Autodesk Fusion 360 part; units mm, degrees
(part 2 of 2)
  line L915 (6.2451, -45) -> (4.5882, -45)
  line L916 (6.2451, 10) -> (4.5882, 10)
  line L917 (3.4167, -7.8284) -> (4.5882, -9)
  line L918 (4.5882, -50) -> (3.4167, -51.1716)
  line L919 (7.4167, -36.1716) -> (6.2451, -35)
  line L920 (3.4167, 13.8284) -> (3.4167, 12.1716)
  line L921 (6.2451, -9) -> (7.4167, -7.8284)
  line L922 (4.5882, -20) -> (3.4167, -21.1716)
  line L923 (4.5882, -10) -> (3.4167, -11.1716)
  line L924 (3.4167, -41.1716) -> (3.4167, -42.8284)
  line L925 (3.4167, 7.1716) -> (4.5882, 6)
  line L926 (4.5882, -15) -> (3.4167, -16.1716)
  line L927 (3.4167, -32.8284) -> (4.5882, -34)
  line L928 (3.4167, -42.8284) -> (4.5882, -44)
  line L929 (6.2451, -25) -> (4.5882, -25)
  line L930 (3.4167, -47.8284) -> (4.5882, -49)
  line L931 (7.4167, -26.1716) -> (6.2451, -25)
  line L932 (4.5882, -39) -> (6.2451, -39)
  line L933 (6.2451, 0) -> (4.5882, 0)
  line L934 (4.5882, 15) -> (3.4167, 13.8284)
  line L935 (3.4167, -37.8284) -> (4.5882, -39)
  line L936 (6.2451, -20) -> (4.5882, -20)
  line L937 (4.5882, 11) -> (6.2451, 11)
  line L938 (7.4167, -11.1716) -> (6.2451, -10)
  line L939 (3.4167, -27.8284) -> (4.5882, -29)
  line L940 (4.5882, 10) -> (3.4167, 8.8284)
  line L941 (6.2451, 11) -> (7.4167, 12.1716)
  line L942 (7.4167, -1.1716) -> (6.2451, 0)
  line L943 (6.2451, -39) -> (7.4167, -37.8284)
  line L944 (4.5882, -45) -> (3.4167, -46.1716)
  line L945 (7.4167, -22.8284) -> (7.4167, -21.1716)
  line L946 (3.4167, -26.1716) -> (3.4167, -27.8284)
  line L947 (3.4167, -16.1716) -> (3.4167, -17.8284)
  line L948 (6.2451, -54) -> (7.4167, -52.8284)
  line L949 (7.4167, -16.1716) -> (6.2451, -15)
  line L950 (3.4167, -11.1716) -> (3.4167, -12.8284)
  line L951 (4.5882, -40) -> (3.4167, -41.1716)
  line L952 (3.4167, -2.8284) -> (4.5882, -4)
  line L953 (3.4167, -12.8284) -> (4.5882, -14)
  line L954 (3.4167, 3.8284) -> (3.4167, 2.1716)
  line L955 (7.4167, -37.8284) -> (7.4167, -36.1716)
  line L956 (7.4167, -52.8284) -> (7.4167, -51.1716)
  line L957 (7.4167, -42.8284) -> (7.4167, -41.1716)
  line L958 (7.4167, 3.8284) -> (6.2451, 5)
  line L959 (6.2451, -5) -> (4.5882, -5)
  line L960 (7.4167, -51.1716) -> (6.2451, -50)
  line L961 (4.5882, -30) -> (3.4167, -31.1716)
  line L962 (4.5882, -4) -> (6.2451, -4)
  line L963 (7.4167, 7.1716) -> (7.4167, 8.8284)
  line L964 (4.5882, -34) -> (6.2451, -34)
  line L965 (6.2451, -15) -> (4.5882, -15)
  line L966 (7.4167, 2.1716) -> (7.4167, 3.8284)
  line L967 (6.2451, 20) -> (4.5882, 20)
  line L968 (4.5882, -54) -> (6.2451, -54)
  line L969 (3.4167, 12.1716) -> (4.5882, 11)
  line L970 (3.4167, -36.1716) -> (3.4167, -37.8284)
  line L971 (7.4167, -41.1716) -> (6.2451, -40)
  line L972 (7.4167, 13.8284) -> (6.2451, 15)
  line L973 (7.4167, 18.8284) -> (6.2451, 20)
  line L974 (7.4167, -7.8284) -> (7.4167, -6.1716)
  line L975 (6.2451, -29) -> (7.4167, -27.8284)
  line L976 (8.3333, -6.1716) -> (8.3333, -7.8284)
  line L977 (11.1618, -40) -> (9.5049, -40)
  line L978 (12.3333, -27.8284) -> (12.3333, -26.1716)
  line L979 (9.5049, 5) -> (8.3333, 3.8284)
  line L980 (8.3333, -31.1716) -> (8.3333, -32.8284)
  line L981 (12.3333, -2.8284) -> (12.3333, -1.1716)
  line L982 (9.5049, 20) -> (8.3333, 18.8284)
  line L983 (8.3333, 2.1716) -> (9.5049, 1)
  line L984 (8.3333, -1.1716) -> (8.3333, -2.8284)
  line L985 (8.3333, 18.8284) -> (8.3333, 17.1716)
  line L986 (9.5049, -29) -> (11.1618, -29)
  line L987 (11.1618, -49) -> (12.3333, -47.8284)
  line L988 (11.1618, 5) -> (9.5049, 5)
  line L989 (11.1618, -24) -> (12.3333, -22.8284)
  line L990 (8.3333, -51.1716) -> (8.3333, -52.8284)
  line L991 (12.3333, -6.1716) -> (11.1618, -5)
  line L992 (12.3333, -47.8284) -> (12.3333, -46.1716)
  line L993 (12.3333, -32.8284) -> (12.3333, -31.1716)
  line L994 (12.3333, 8.8284) -> (11.1618, 10)
  line L995 (8.3333, 17.1716) -> (9.5049, 16)
  line L996 (9.5049, -9) -> (11.1618, -9)
  line L997 (12.3333, -46.1716) -> (11.1618, -45)
  line L998 (11.1618, 16) -> (12.3333, 17.1716)
  line L999 (11.1618, -44) -> (12.3333, -42.8284)
  line L1000 (9.5049, -14) -> (11.1618, -14)
  line L1001 (11.1618, 6) -> (12.3333, 7.1716)
  line L1002 (9.5049, -49) -> (11.1618, -49)
  line L1003 (9.5049, -44) -> (11.1618, -44)
  line L1004 (12.3333, -21.1716) -> (11.1618, -20)
  line L1005 (9.5049, 1) -> (11.1618, 1)
  line L1006 (11.1618, -4) -> (12.3333, -2.8284)
  line L1007 (12.3333, -17.8284) -> (12.3333, -16.1716)
  line L1008 (11.1618, -30) -> (9.5049, -30)
  line L1009 (9.5049, -5) -> (8.3333, -6.1716)
  line L1010 (11.1618, -19) -> (12.3333, -17.8284)
  line L1011 (11.1618, -14) -> (12.3333, -12.8284)
  line L1012 (8.3333, -22.8284) -> (9.5049, -24)
  line L1013 (11.1618, -34) -> (12.3333, -32.8284)
  line L1014 (12.3333, -31.1716) -> (11.1618, -30)
  line L1015 (12.3333, -12.8284) -> (12.3333, -11.1716)
  line L1016 (8.3333, -21.1716) -> (8.3333, -22.8284)
  line L1017 (9.5049, -35) -> (8.3333, -36.1716)
  line L1018 (9.5049, 0) -> (8.3333, -1.1716)
  line L1019 (8.3333, -52.8284) -> (9.5049, -54)
  line L1020 (11.1618, -10) -> (9.5049, -10)
  line L1021 (11.1618, 1) -> (12.3333, 2.1716)
  line L1022 (8.3333, -17.8284) -> (9.5049, -19)
  line L1023 (8.3333, -46.1716) -> (8.3333, -47.8284)
  line L1024 (12.3333, 17.1716) -> (12.3333, 18.8284)
  line L1025 (9.5049, -19) -> (11.1618, -19)
  line L1026 (9.5049, 16) -> (11.1618, 16)
  line L1027 (9.5049, 6) -> (11.1618, 6)
  line L1028 (9.5049, -24) -> (11.1618, -24)
  line L1029 (9.5049, -25) -> (8.3333, -26.1716)
  line L1030 (11.1618, -35) -> (9.5049, -35)
  line L1031 (12.3333, 12.1716) -> (12.3333, 13.8284)
  line L1032 (11.1618, -50) -> (9.5049, -50)
  line L1033 (8.3333, 8.8284) -> (8.3333, 7.1716)
  line L1034 (11.1618, 15) -> (9.5049, 15)
  line L1035 (11.1618, -45) -> (9.5049, -45)
  line L1036 (11.1618, 10) -> (9.5049, 10)
  line L1037 (8.3333, -7.8284) -> (9.5049, -9)
  line L1038 (9.5049, -50) -> (8.3333, -51.1716)
  line L1039 (12.3333, -36.1716) -> (11.1618, -35)
  line L1040 (8.3333, 13.8284) -> (8.3333, 12.1716)
  line L1041 (11.1618, -9) -> (12.3333, -7.8284)
  line L1042 (9.5049, -20) -> (8.3333, -21.1716)
  line L1043 (9.5049, -10) -> (8.3333, -11.1716)
  line L1044 (8.3333, -41.1716) -> (8.3333, -42.8284)
  line L1045 (8.3333, 7.1716) -> (9.5049, 6)
  line L1046 (9.5049, -15) -> (8.3333, -16.1716)
  line L1047 (8.3333, -32.8284) -> (9.5049, -34)
  line L1048 (8.3333, -42.8284) -> (9.5049, -44)
  line L1049 (11.1618, -25) -> (9.5049, -25)
  line L1050 (8.3333, -47.8284) -> (9.5049, -49)
  line L1051 (12.3333, -26.1716) -> (11.1618, -25)
  line L1052 (9.5049, -39) -> (11.1618, -39)
  line L1053 (11.1618, 0) -> (9.5049, 0)
  line L1054 (9.5049, 15) -> (8.3333, 13.8284)
  line L1055 (8.3333, -37.8284) -> (9.5049, -39)
  line L1056 (11.1618, -20) -> (9.5049, -20)
  line L1057 (9.5049, 11) -> (11.1618, 11)
  line L1058 (12.3333, -11.1716) -> (11.1618, -10)
  line L1059 (8.3333, -27.8284) -> (9.5049, -29)
  line L1060 (9.5049, 10) -> (8.3333, 8.8284)
  line L1061 (11.1618, 11) -> (12.3333, 12.1716)
  line L1062 (12.3333, -1.1716) -> (11.1618, 0)
  line L1063 (11.1618, -39) -> (12.3333, -37.8284)
  line L1064 (9.5049, -45) -> (8.3333, -46.1716)
  line L1065 (12.3333, -22.8284) -> (12.3333, -21.1716)
  line L1066 (8.3333, -26.1716) -> (8.3333, -27.8284)
  line L1067 (8.3333, -16.1716) -> (8.3333, -17.8284)
  line L1068 (11.1618, -54) -> (12.3333, -52.8284)
  line L1069 (12.3333, -16.1716) -> (11.1618, -15)
  line L1070 (8.3333, -11.1716) -> (8.3333, -12.8284)
  line L1071 (9.5049, -40) -> (8.3333, -41.1716)
  line L1072 (8.3333, -2.8284) -> (9.5049, -4)
  line L1073 (8.3333, -12.8284) -> (9.5049, -14)
  line L1074 (8.3333, 3.8284) -> (8.3333, 2.1716)
  line L1075 (12.3333, -37.8284) -> (12.3333, -36.1716)
  line L1076 (12.3333, -52.8284) -> (12.3333, -51.1716)
  line L1077 (12.3333, -42.8284) -> (12.3333, -41.1716)
  line L1078 (12.3333, 3.8284) -> (11.1618, 5)
  line L1079 (11.1618, -5) -> (9.5049, -5)
  line L1080 (12.3333, -51.1716) -> (11.1618, -50)
  line L1081 (9.5049, -30) -> (8.3333, -31.1716)
  line L1082 (9.5049, -4) -> (11.1618, -4)
  line L1083 (12.3333, 7.1716) -> (12.3333, 8.8284)
  line L1084 (9.5049, -34) -> (11.1618, -34)
  line L1085 (11.1618, -15) -> (9.5049, -15)
  line L1086 (12.3333, 2.1716) -> (12.3333, 3.8284)
  line L1087 (11.1618, 20) -> (9.5049, 20)
  line L1088 (9.5049, -54) -> (11.1618, -54)
  line L1089 (8.3333, 12.1716) -> (9.5049, 11)
  line L1090 (8.3333, -36.1716) -> (8.3333, -37.8284)
  line L1091 (12.3333, -41.1716) -> (11.1618, -40)
  line L1092 (12.3333, 13.8284) -> (11.1618, 15)
  line L1093 (12.3333, 18.8284) -> (11.1618, 20)
  line L1094 (12.3333, -7.8284) -> (12.3333, -6.1716)
  line L1095 (11.1618, -29) -> (12.3333, -27.8284)
  line L1096 (13.25, -6.1716) -> (13.25, -7.8284)
  line L1097 (16.0784, -40) -> (14.4216, -40)
  line L1098 (17.25, -27.8284) -> (17.25, -26.1716)
  line L1099 (14.4216, 5) -> (13.25, 3.8284)
  line L1100 (13.25, -31.1716) -> (13.25, -32.8284)
  line L1101 (17.25, -2.8284) -> (17.25, -1.1716)
  line L1102 (14.4216, 20) -> (13.25, 18.8284)
  line L1103 (13.25, 2.1716) -> (14.4216, 1)
  line L1104 (13.25, -1.1716) -> (13.25, -2.8284)
  line L1105 (13.25, 18.8284) -> (13.25, 17.1716)
  line L1106 (14.4216, -29) -> (16.0784, -29)
  line L1107 (16.0784, -49) -> (17.25, -47.8284)
  line L1108 (16.0784, 5) -> (14.4216, 5)
  line L1109 (16.0784, -24) -> (17.25, -22.8284)
  line L1110 (13.25, -51.1716) -> (13.25, -52.8284)
  line L1111 (17.25, -6.1716) -> (16.0784, -5)
  line L1112 (17.25, -47.8284) -> (17.25, -46.1716)
  line L1113 (17.25, -32.8284) -> (17.25, -31.1716)
  line L1114 (17.25, 8.8284) -> (16.0784, 10)
  line L1115 (13.25, 17.1716) -> (14.4216, 16)
  line L1116 (14.4216, -9) -> (16.0784, -9)
  line L1117 (17.25, -46.1716) -> (16.0784, -45)
  line L1118 (16.0784, 16) -> (17.25, 17.1716)
  line L1119 (16.0784, -44) -> (17.25, -42.8284)
  line L1120 (14.4216, -14) -> (16.0784, -14)
  line L1121 (16.0784, 6) -> (17.25, 7.1716)
  line L1122 (14.4216, -49) -> (16.0784, -49)
  line L1123 (14.4216, -44) -> (16.0784, -44)
  line L1124 (17.25, -21.1716) -> (16.0784, -20)
  line L1125 (14.4216, 1) -> (16.0784, 1)
  line L1126 (16.0784, -4) -> (17.25, -2.8284)
  line L1127 (17.25, -17.8284) -> (17.25, -16.1716)
  line L1128 (16.0784, -30) -> (14.4216, -30)
  line L1129 (14.4216, -5) -> (13.25, -6.1716)
  line L1130 (16.0784, -19) -> (17.25, -17.8284)
  line L1131 (16.0784, -14) -> (17.25, -12.8284)
  line L1132 (13.25, -22.8284) -> (14.4216, -24)
  line L1133 (16.0784, -34) -> (17.25, -32.8284)
  line L1134 (17.25, -31.1716) -> (16.0784, -30)
  line L1135 (17.25, -12.8284) -> (17.25, -11.1716)
  line L1136 (13.25, -21.1716) -> (13.25, -22.8284)
  line L1137 (14.4216, -35) -> (13.25, -36.1716)
  line L1138 (14.4216, 0) -> (13.25, -1.1716)
  line L1139 (13.25, -52.8284) -> (14.4216, -54)
  line L1140 (16.0784, -10) -> (14.4216, -10)
  line L1141 (16.0784, 1) -> (17.25, 2.1716)
  line L1142 (13.25, -17.8284) -> (14.4216, -19)
  line L1143 (13.25, -46.1716) -> (13.25, -47.8284)
  line L1144 (17.25, 17.1716) -> (17.25, 18.8284)
  line L1145 (14.4216, -19) -> (16.0784, -19)
  line L1146 (14.4216, 16) -> (16.0784, 16)
  line L1147 (14.4216, 6) -> (16.0784, 6)
  line L1148 (14.4216, -24) -> (16.0784, -24)
  line L1149 (14.4216, -25) -> (13.25, -26.1716)
  line L1150 (16.0784, -35) -> (14.4216, -35)
  line L1151 (17.25, 12.1716) -> (17.25, 13.8284)
  line L1152 (16.0784, -50) -> (14.4216, -50)
  line L1153 (13.25, 8.8284) -> (13.25, 7.1716)
  line L1154 (16.0784, 15) -> (14.4216, 15)
  line L1155 (16.0784, -45) -> (14.4216, -45)
  line L1156 (16.0784, 10) -> (14.4216, 10)
  line L1157 (13.25, -7.8284) -> (14.4216, -9)
  line L1158 (14.4216, -50) -> (13.25, -51.1716)
  line L1159 (17.25, -36.1716) -> (16.0784, -35)
  line L1160 (13.25, 13.8284) -> (13.25, 12.1716)
  line L1161 (16.0784, -9) -> (17.25, -7.8284)
  line L1162 (14.4216, -20) -> (13.25, -21.1716)
  line L1163 (14.4216, -10) -> (13.25, -11.1716)
  line L1164 (13.25, -41.1716) -> (13.25, -42.8284)
  line L1165 (13.25, 7.1716) -> (14.4216, 6)
  line L1166 (14.4216, -15) -> (13.25, -16.1716)
  line L1167 (13.25, -32.8284) -> (14.4216, -34)
  line L1168 (13.25, -42.8284) -> (14.4216, -44)
  line L1169 (16.0784, -25) -> (14.4216, -25)
  line L1170 (13.25, -47.8284) -> (14.4216, -49)
  line L1171 (17.25, -26.1716) -> (16.0784, -25)
  line L1172 (14.4216, -39) -> (16.0784, -39)
  line L1173 (16.0784, 0) -> (14.4216, 0)
  line L1174 (14.4216, 15) -> (13.25, 13.8284)
  line L1175 (13.25, -37.8284) -> (14.4216, -39)
  line L1176 (16.0784, -20) -> (14.4216, -20)
  line L1177 (14.4216, 11) -> (16.0784, 11)
  line L1178 (17.25, -11.1716) -> (16.0784, -10)
  line L1179 (13.25, -27.8284) -> (14.4216, -29)
  line L1180 (14.4216, 10) -> (13.25, 8.8284)
  line L1181 (16.0784, 11) -> (17.25, 12.1716)
  line L1182 (17.25, -1.1716) -> (16.0784, 0)
  line L1183 (16.0784, -39) -> (17.25, -37.8284)
  line L1184 (14.4216, -45) -> (13.25, -46.1716)
  line L1185 (17.25, -22.8284) -> (17.25, -21.1716)
  line L1186 (13.25, -26.1716) -> (13.25, -27.8284)
  line L1187 (13.25, -16.1716) -> (13.25, -17.8284)
  line L1188 (16.0784, -54) -> (17.25, -52.8284)
  line L1189 (17.25, -16.1716) -> (16.0784, -15)
  line L1190 (13.25, -11.1716) -> (13.25, -12.8284)
  line L1191 (14.4216, -40) -> (13.25, -41.1716)
  line L1192 (13.25, -2.8284) -> (14.4216, -4)
  line L1193 (13.25, -12.8284) -> (14.4216, -14)
  line L1194 (13.25, 3.8284) -> (13.25, 2.1716)
  line L1195 (17.25, -37.8284) -> (17.25, -36.1716)
  line L1196 (17.25, -52.8284) -> (17.25, -51.1716)
  line L1197 (17.25, -42.8284) -> (17.25, -41.1716)
  line L1198 (17.25, 3.8284) -> (16.0784, 5)
  line L1199 (16.0784, -5) -> (14.4216, -5)
  line L1200 (17.25, -51.1716) -> (16.0784, -50)
  line L1201 (14.4216, -30) -> (13.25, -31.1716)
  line L1202 (14.4216, -4) -> (16.0784, -4)
  line L1203 (17.25, 7.1716) -> (17.25, 8.8284)
  line L1204 (14.4216, -34) -> (16.0784, -34)
  line L1205 (16.0784, -15) -> (14.4216, -15)
  line L1206 (17.25, 2.1716) -> (17.25, 3.8284)
  line L1207 (16.0784, 20) -> (14.4216, 20)
  line L1208 (14.4216, -54) -> (16.0784, -54)
  line L1209 (13.25, 12.1716) -> (14.4216, 11)
  line L1210 (13.25, -36.1716) -> (13.25, -37.8284)
  line L1211 (17.25, -41.1716) -> (16.0784, -40)
  line L1212 (17.25, 13.8284) -> (16.0784, 15)
  line L1213 (17.25, 18.8284) -> (16.0784, 20)
  line L1214 (17.25, -7.8284) -> (17.25, -6.1716)
  line L1215 (16.0784, -29) -> (17.25, -27.8284)
  line L1216 (18.1667, -6.1716) -> (18.1667, -7.8284)
  line L1217 (20.9951, -40) -> (19.3382, -40)
  line L1218 (22.1667, -27.8284) -> (22.1667, -26.1716)
  line L1219 (19.3382, 5) -> (18.1667, 3.8284)
  line L1220 (18.1667, -31.1716) -> (18.1667, -32.8284)
  line L1221 (22.1667, -2.8284) -> (22.1667, -1.1716)
  line L1222 (19.3382, 20) -> (18.1667, 18.8284)
  line L1223 (18.1667, 2.1716) -> (19.3382, 1)
  line L1224 (18.1667, -1.1716) -> (18.1667, -2.8284)
  line L1225 (18.1667, 18.8284) -> (18.1667, 17.1716)
  line L1226 (19.3382, -29) -> (20.9951, -29)
  line L1227 (20.9951, -49) -> (22.1667, -47.8284)
  line L1228 (20.9951, 5) -> (19.3382, 5)
  line L1229 (20.9951, -24) -> (22.1667, -22.8284)
  line L1230 (18.1667, -51.1716) -> (18.1667, -52.8284)
  line L1231 (22.1667, -6.1716) -> (20.9951, -5)
  line L1232 (22.1667, -47.8284) -> (22.1667, -46.1716)
  line L1233 (22.1667, -32.8284) -> (22.1667, -31.1716)
  line L1234 (22.1667, 8.8284) -> (20.9951, 10)
  line L1235 (18.1667, 17.1716) -> (19.3382, 16)
  line L1236 (19.3382, -9) -> (20.9951, -9)
  line L1237 (22.1667, -46.1716) -> (20.9951, -45)
  line L1238 (20.9951, 16) -> (22.1667, 17.1716)
  line L1239 (20.9951, -44) -> (22.1667, -42.8284)
  line L1240 (19.3382, -14) -> (20.9951, -14)
  line L1241 (20.9951, 6) -> (22.1667, 7.1716)
  line L1242 (19.3382, -49) -> (20.9951, -49)
  line L1243 (19.3382, -44) -> (20.9951, -44)
  line L1244 (22.1667, -21.1716) -> (20.9951, -20)
  line L1245 (19.3382, 1) -> (20.9951, 1)
  line L1246 (20.9951, -4) -> (22.1667, -2.8284)
  line L1247 (22.1667, -17.8284) -> (22.1667, -16.1716)
  line L1248 (20.9951, -30) -> (19.3382, -30)
  line L1249 (19.3382, -5) -> (18.1667, -6.1716)
  line L1250 (20.9951, -19) -> (22.1667, -17.8284)
  line L1251 (20.9951, -14) -> (22.1667, -12.8284)
  line L1252 (18.1667, -22.8284) -> (19.3382, -24)
  line L1253 (20.9951, -34) -> (22.1667, -32.8284)
  line L1254 (22.1667, -31.1716) -> (20.9951, -30)
  line L1255 (22.1667, -12.8284) -> (22.1667, -11.1716)
  line L1256 (18.1667, -21.1716) -> (18.1667, -22.8284)
  line L1257 (19.3382, -35) -> (18.1667, -36.1716)
  line L1258 (19.3382, 0) -> (18.1667, -1.1716)
  line L1259 (18.1667, -52.8284) -> (19.3382, -54)
  line L1260 (20.9951, -10) -> (19.3382, -10)
  line L1261 (20.9951, 1) -> (22.1667, 2.1716)
  line L1262 (18.1667, -17.8284) -> (19.3382, -19)
  line L1263 (18.1667, -46.1716) -> (18.1667, -47.8284)
  line L1264 (22.1667, 17.1716) -> (22.1667, 18.8284)
  line L1265 (19.3382, -19) -> (20.9951, -19)
  line L1266 (19.3382, 16) -> (20.9951, 16)
  line L1267 (19.3382, 6) -> (20.9951, 6)
  line L1268 (19.3382, -24) -> (20.9951, -24)
  line L1269 (19.3382, -25) -> (18.1667, -26.1716)
  line L1270 (20.9951, -35) -> (19.3382, -35)
  line L1271 (22.1667, 12.1716) -> (22.1667, 13.8284)
  line L1272 (20.9951, -50) -> (19.3382, -50)
  line L1273 (18.1667, 8.8284) -> (18.1667, 7.1716)
  line L1274 (20.9951, 15) -> (19.3382, 15)
  line L1275 (20.9951, -45) -> (19.3382, -45)
  line L1276 (20.9951, 10) -> (19.3382, 10)
  line L1277 (18.1667, -7.8284) -> (19.3382, -9)
  line L1278 (19.3382, -50) -> (18.1667, -51.1716)
  line L1279 (22.1667, -36.1716) -> (20.9951, -35)
  line L1280 (18.1667, 13.8284) -> (18.1667, 12.1716)
  line L1281 (20.9951, -9) -> (22.1667, -7.8284)
  line L1282 (19.3382, -20) -> (18.1667, -21.1716)
  line L1283 (19.3382, -10) -> (18.1667, -11.1716)
  line L1284 (18.1667, -41.1716) -> (18.1667, -42.8284)
  line L1285 (18.1667, 7.1716) -> (19.3382, 6)
  line L1286 (19.3382, -15) -> (18.1667, -16.1716)
  line L1287 (18.1667, -32.8284) -> (19.3382, -34)
  line L1288 (18.1667, -42.8284) -> (19.3382, -44)
  line L1289 (20.9951, -25) -> (19.3382, -25)
  line L1290 (18.1667, -47.8284) -> (19.3382, -49)
  line L1291 (22.1667, -26.1716) -> (20.9951, -25)
  line L1292 (19.3382, -39) -> (20.9951, -39)
  line L1293 (20.9951, 0) -> (19.3382, 0)
  line L1294 (19.3382, 15) -> (18.1667, 13.8284)
  line L1295 (18.1667, -37.8284) -> (19.3382, -39)
  line L1296 (20.9951, -20) -> (19.3382, -20)
  line L1297 (19.3382, 11) -> (20.9951, 11)
  line L1298 (22.1667, -11.1716) -> (20.9951, -10)
  line L1299 (18.1667, -27.8284) -> (19.3382, -29)
  line L1300 (19.3382, 10) -> (18.1667, 8.8284)
  line L1301 (20.9951, 11) -> (22.1667, 12.1716)
  line L1302 (22.1667, -1.1716) -> (20.9951, 0)
  line L1303 (20.9951, -39) -> (22.1667, -37.8284)
  line L1304 (19.3382, -45) -> (18.1667, -46.1716)
  line L1305 (22.1667, -22.8284) -> (22.1667, -21.1716)
  line L1306 (18.1667, -26.1716) -> (18.1667, -27.8284)
  line L1307 (18.1667, -16.1716) -> (18.1667, -17.8284)
  line L1308 (20.9951, -54) -> (22.1667, -52.8284)
  line L1309 (22.1667, -16.1716) -> (20.9951, -15)
  line L1310 (18.1667, -11.1716) -> (18.1667, -12.8284)
  line L1311 (19.3382, -40) -> (18.1667, -41.1716)
  line L1312 (18.1667, -2.8284) -> (19.3382, -4)
  line L1313 (18.1667, -12.8284) -> (19.3382, -14)
  line L1314 (18.1667, 3.8284) -> (18.1667, 2.1716)
  line L1315 (22.1667, -37.8284) -> (22.1667, -36.1716)
  line L1316 (22.1667, -52.8284) -> (22.1667, -51.1716)
  line L1317 (22.1667, -42.8284) -> (22.1667, -41.1716)
  line L1318 (22.1667, 3.8284) -> (20.9951, 5)
  line L1319 (20.9951, -5) -> (19.3382, -5)
  line L1320 (22.1667, -51.1716) -> (20.9951, -50)
  line L1321 (19.3382, -30) -> (18.1667, -31.1716)
  line L1322 (19.3382, -4) -> (20.9951, -4)
  line L1323 (22.1667, 7.1716) -> (22.1667, 8.8284)
  line L1324 (19.3382, -34) -> (20.9951, -34)
  line L1325 (20.9951, -15) -> (19.3382, -15)
  line L1326 (22.1667, 2.1716) -> (22.1667, 3.8284)
  line L1327 (20.9951, 20) -> (19.3382, 20)
  line L1328 (19.3382, -54) -> (20.9951, -54)
  line L1329 (18.1667, 12.1716) -> (19.3382, 11)
  line L1330 (18.1667, -36.1716) -> (18.1667, -37.8284)
  line L1331 (22.1667, -41.1716) -> (20.9951, -40)
  line L1332 (22.1667, 13.8284) -> (20.9951, 15)
  line L1333 (22.1667, 18.8284) -> (20.9951, 20)
  line L1334 (22.1667, -7.8284) -> (22.1667, -6.1716)
  line L1335 (20.9951, -29) -> (22.1667, -27.8284)
  line L1336 (23.0833, -6.1716) -> (23.0833, -7.8284)
  line L1337 (25.9118, -40) -> (24.2549, -40)
  line L1338 (27.0833, -27.8284) -> (27.0833, -26.1716)
  line L1339 (24.2549, 5) -> (23.0833, 3.8284)
  line L1340 (23.0833, -31.1716) -> (23.0833, -32.8284)
  line L1341 (27.0833, -2.8284) -> (27.0833, -1.1716)
  line L1342 (24.2549, 20) -> (23.0833, 18.8284)
  line L1343 (23.0833, 2.1716) -> (24.2549, 1)
  line L1344 (23.0833, -1.1716) -> (23.0833, -2.8284)
  line L1345 (23.0833, 18.8284) -> (23.0833, 17.1716)
  line L1346 (24.2549, -29) -> (25.9118, -29)
  line L1347 (25.9118, -49) -> (27.0833, -47.8284)
  line L1348 (25.9118, 5) -> (24.2549, 5)
  line L1349 (25.9118, -24) -> (27.0833, -22.8284)
  line L1350 (23.0833, -51.1716) -> (23.0833, -52.8284)
  line L1351 (27.0833, -6.1716) -> (25.9118, -5)
  line L1352 (27.0833, -47.8284) -> (27.0833, -46.1716)
  line L1353 (27.0833, -32.8284) -> (27.0833, -31.1716)
  line L1354 (27.0833, 8.8284) -> (25.9118, 10)
  line L1355 (23.0833, 17.1716) -> (24.2549, 16)
  line L1356 (24.2549, -9) -> (25.9118, -9)
  line L1357 (27.0833, -46.1716) -> (25.9118, -45)
  line L1358 (25.9118, 16) -> (27.0833, 17.1716)
  line L1359 (25.9118, -44) -> (27.0833, -42.8284)
  line L1360 (24.2549, -14) -> (25.9118, -14)
  line L1361 (25.9118, 6) -> (27.0833, 7.1716)
  line L1362 (24.2549, -49) -> (25.9118, -49)
  line L1363 (24.2549, -44) -> (25.9118, -44)
  line L1364 (27.0833, -21.1716) -> (25.9118, -20)
  line L1365 (24.2549, 1) -> (25.9118, 1)
  line L1366 (25.9118, -4) -> (27.0833, -2.8284)
  line L1367 (27.0833, -17.8284) -> (27.0833, -16.1716)
  line L1368 (25.9118, -30) -> (24.2549, -30)
  line L1369 (24.2549, -5) -> (23.0833, -6.1716)
  line L1370 (25.9118, -19) -> (27.0833, -17.8284)
  line L1371 (25.9118, -14) -> (27.0833, -12.8284)
  line L1372 (23.0833, -22.8284) -> (24.2549, -24)
  line L1373 (25.9118, -34) -> (27.0833, -32.8284)
  line L1374 (27.0833, -31.1716) -> (25.9118, -30)
  line L1375 (27.0833, -12.8284) -> (27.0833, -11.1716)
  line L1376 (23.0833, -21.1716) -> (23.0833, -22.8284)
  line L1377 (24.2549, -35) -> (23.0833, -36.1716)
  line L1378 (24.2549, 0) -> (23.0833, -1.1716)
  line L1379 (23.0833, -52.8284) -> (24.2549, -54)
  line L1380 (25.9118, -10) -> (24.2549, -10)
  line L1381 (25.9118, 1) -> (27.0833, 2.1716)
  line L1382 (23.0833, -17.8284) -> (24.2549, -19)
  line L1383 (23.0833, -46.1716) -> (23.0833, -47.8284)
  line L1384 (27.0833, 17.1716) -> (27.0833, 18.8284)
  line L1385 (24.2549, -19) -> (25.9118, -19)
  line L1386 (24.2549, 16) -> (25.9118, 16)
  line L1387 (24.2549, 6) -> (25.9118, 6)
  line L1388 (24.2549, -24) -> (25.9118, -24)
  line L1389 (24.2549, -25) -> (23.0833, -26.1716)
  line L1390 (25.9118, -35) -> (24.2549, -35)
  line L1391 (27.0833, 12.1716) -> (27.0833, 13.8284)
  line L1392 (25.9118, -50) -> (24.2549, -50)
  line L1393 (23.0833, 8.8284) -> (23.0833, 7.1716)
  line L1394 (25.9118, 15) -> (24.2549, 15)
  line L1395 (25.9118, -45) -> (24.2549, -45)
  line L1396 (25.9118, 10) -> (24.2549, 10)
  line L1397 (23.0833, -7.8284) -> (24.2549, -9)
  line L1398 (24.2549, -50) -> (23.0833, -51.1716)
  line L1399 (27.0833, -36.1716) -> (25.9118, -35)
  line L1400 (23.0833, 13.8284) -> (23.0833, 12.1716)
  line L1401 (25.9118, -9) -> (27.0833, -7.8284)
  line L1402 (24.2549, -20) -> (23.0833, -21.1716)
  line L1403 (24.2549, -10) -> (23.0833, -11.1716)
  line L1404 (23.0833, -41.1716) -> (23.0833, -42.8284)
  line L1405 (23.0833, 7.1716) -> (24.2549, 6)
  line L1406 (24.2549, -15) -> (23.0833, -16.1716)
  line L1407 (23.0833, -32.8284) -> (24.2549, -34)
  line L1408 (23.0833, -42.8284) -> (24.2549, -44)
  line L1409 (25.9118, -25) -> (24.2549, -25)
  line L1410 (23.0833, -47.8284) -> (24.2549, -49)
  line L1411 (27.0833, -26.1716) -> (25.9118, -25)
  line L1412 (24.2549, -39) -> (25.9118, -39)
  line L1413 (25.9118, 0) -> (24.2549, 0)
  line L1414 (24.2549, 15) -> (23.0833, 13.8284)
  line L1415 (23.0833, -37.8284) -> (24.2549, -39)
  line L1416 (25.9118, -20) -> (24.2549, -20)
  line L1417 (24.2549, 11) -> (25.9118, 11)
  line L1418 (27.0833, -11.1716) -> (25.9118, -10)
  line L1419 (23.0833, -27.8284) -> (24.2549, -29)
  line L1420 (24.2549, 10) -> (23.0833, 8.8284)
  line L1421 (25.9118, 11) -> (27.0833, 12.1716)
  line L1422 (27.0833, -1.1716) -> (25.9118, 0)
  line L1423 (25.9118, -39) -> (27.0833, -37.8284)
  line L1424 (24.2549, -45) -> (23.0833, -46.1716)
  line L1425 (27.0833, -22.8284) -> (27.0833, -21.1716)
  line L1426 (23.0833, -26.1716) -> (23.0833, -27.8284)
  line L1427 (23.0833, -16.1716) -> (23.0833, -17.8284)
  line L1428 (25.9118, -54) -> (27.0833, -52.8284)
  line L1429 (27.0833, -16.1716) -> (25.9118, -15)
  line L1430 (23.0833, -11.1716) -> (23.0833, -12.8284)
  line L1431 (24.2549, -40) -> (23.0833, -41.1716)
  line L1432 (23.0833, -2.8284) -> (24.2549, -4)
  line L1433 (23.0833, -12.8284) -> (24.2549, -14)
  line L1434 (23.0833, 3.8284) -> (23.0833, 2.1716)
  line L1435 (27.0833, -37.8284) -> (27.0833, -36.1716)
  line L1436 (27.0833, -52.8284) -> (27.0833, -51.1716)
  line L1437 (27.0833, -42.8284) -> (27.0833, -41.1716)
  line L1438 (27.0833, 3.8284) -> (25.9118, 5)
  line L1439 (25.9118, -5) -> (24.2549, -5)
  line L1440 (27.0833, -51.1716) -> (25.9118, -50)
  line L1441 (24.2549, -30) -> (23.0833, -31.1716)
  line L1442 (24.2549, -4) -> (25.9118, -4)
  line L1443 (27.0833, 7.1716) -> (27.0833, 8.8284)
  line L1444 (24.2549, -34) -> (25.9118, -34)
  line L1445 (25.9118, -15) -> (24.2549, -15)
  line L1446 (27.0833, 2.1716) -> (27.0833, 3.8284)
  line L1447 (25.9118, 20) -> (24.2549, 20)
  line L1448 (24.2549, -54) -> (25.9118, -54)
  line L1449 (23.0833, 12.1716) -> (24.2549, 11)
  line L1450 (23.0833, -36.1716) -> (23.0833, -37.8284)
  line L1451 (27.0833, -41.1716) -> (25.9118, -40)
  line L1452 (27.0833, 13.8284) -> (25.9118, 15)
  line L1453 (27.0833, 18.8284) -> (25.9118, 20)
  line L1454 (27.0833, -7.8284) -> (27.0833, -6.1716)
  line L1455 (25.9118, -29) -> (27.0833, -27.8284)
  line L1456 (28, -6.1716) -> (28, -7.8284)
  line L1457 (30.8284, -40) -> (29.1716, -40)
  line L1458 (32, -27.8284) -> (32, -26.1716)
  line L1459 (29.1716, 5) -> (28, 3.8284)
  line L1460 (28, -31.1716) -> (28, -32.8284)
  line L1461 (32, -2.8284) -> (32, -1.1716)
  line L1462 (29.1716, 20) -> (28, 18.8284)
  line L1463 (28, 2.1716) -> (29.1716, 1)
  line L1464 (28, -1.1716) -> (28, -2.8284)
  line L1465 (28, 18.8284) -> (28, 17.1716)
  line L1466 (29.1716, -29) -> (30.8284, -29)
  line L1467 (30.8284, -49) -> (32, -47.8284)
  line L1468 (30.8284, 5) -> (29.1716, 5)
  line L1469 (30.8284, -24) -> (32, -22.8284)
  line L1470 (28, -51.1716) -> (28, -52.8284)
  line L1471 (32, -6.1716) -> (30.8284, -5)
  line L1472 (32, -47.8284) -> (32, -46.1716)
  line L1473 (32, -32.8284) -> (32, -31.1716)
  line L1474 (32, 8.8284) -> (30.8284, 10)
  line L1475 (28, 17.1716) -> (29.1716, 16)
  line L1476 (29.1716, -9) -> (30.8284, -9)
  line L1477 (32, -46.1716) -> (30.8284, -45)
  line L1478 (30.8284, 16) -> (32, 17.1716)
  line L1479 (30.8284, -44) -> (32, -42.8284)
  line L1480 (29.1716, -14) -> (30.8284, -14)
  line L1481 (30.8284, 6) -> (32, 7.1716)
  line L1482 (29.1716, -49) -> (30.8284, -49)
  line L1483 (29.1716, -44) -> (30.8284, -44)
  line L1484 (32, -21.1716) -> (30.8284, -20)
  line L1485 (29.1716, 1) -> (30.8284, 1)
  line L1486 (30.8284, -4) -> (32, -2.8284)
  line L1487 (32, -17.8284) -> (32, -16.1716)
  line L1488 (30.8284, -30) -> (29.1716, -30)
  line L1489 (29.1716, -5) -> (28, -6.1716)
  line L1490 (30.8284, -19) -> (32, -17.8284)
  line L1491 (30.8284, -14) -> (32, -12.8284)
  line L1492 (28, -22.8284) -> (29.1716, -24)
  line L1493 (30.8284, -34) -> (32, -32.8284)
  line L1494 (32, -31.1716) -> (30.8284, -30)
  line L1495 (32, -12.8284) -> (32, -11.1716)
  line L1496 (28, -21.1716) -> (28, -22.8284)
  line L1497 (29.1716, -35) -> (28, -36.1716)
  line L1498 (29.1716, 0) -> (28, -1.1716)
  line L1499 (28, -52.8284) -> (29.1716, -54)
  line L1500 (30.8284, -10) -> (29.1716, -10)
  line L1501 (30.8284, 1) -> (32, 2.1716)
  line L1502 (28, -17.8284) -> (29.1716, -19)
  line L1503 (28, -46.1716) -> (28, -47.8284)
  line L1504 (32, 17.1716) -> (32, 18.8284)
  line L1505 (29.1716, -19) -> (30.8284, -19)
  line L1506 (29.1716, 16) -> (30.8284, 16)
  line L1507 (29.1716, 6) -> (30.8284, 6)
  line L1508 (29.1716, -24) -> (30.8284, -24)
  line L1509 (29.1716, -25) -> (28, -26.1716)
  line L1510 (30.8284, -35) -> (29.1716, -35)
  line L1511 (32, 12.1716) -> (32, 13.8284)
  line L1512 (30.8284, -50) -> (29.1716, -50)
  line L1513 (28, 8.8284) -> (28, 7.1716)
  line L1514 (30.8284, 15) -> (29.1716, 15)
  line L1515 (30.8284, -45) -> (29.1716, -45)
  line L1516 (30.8284, 10) -> (29.1716, 10)
  line L1517 (28, -7.8284) -> (29.1716, -9)
  line L1518 (29.1716, -50) -> (28, -51.1716)
  line L1519 (32, -36.1716) -> (30.8284, -35)
  line L1520 (28, 13.8284) -> (28, 12.1716)
  line L1521 (30.8284, -9) -> (32, -7.8284)
  line L1522 (29.1716, -20) -> (28, -21.1716)
  line L1523 (29.1716, -10) -> (28, -11.1716)
  line L1524 (28, -41.1716) -> (28, -42.8284)
  line L1525 (28, 7.1716) -> (29.1716, 6)
  line L1526 (29.1716, -15) -> (28, -16.1716)
  line L1527 (28, -32.8284) -> (29.1716, -34)
  line L1528 (28, -42.8284) -> (29.1716, -44)
  line L1529 (30.8284, -25) -> (29.1716, -25)
  line L1530 (28, -47.8284) -> (29.1716, -49)
  line L1531 (32, -26.1716) -> (30.8284, -25)
  line L1532 (29.1716, -39) -> (30.8284, -39)
  line L1533 (30.8284, 0) -> (29.1716, 0)
  line L1534 (29.1716, 15) -> (28, 13.8284)
  line L1535 (28, -37.8284) -> (29.1716, -39)
  line L1536 (30.8284, -20) -> (29.1716, -20)
  line L1537 (29.1716, 11) -> (30.8284, 11)
  line L1538 (32, -11.1716) -> (30.8284, -10)
  line L1539 (28, -27.8284) -> (29.1716, -29)
  line L1540 (29.1716, 10) -> (28, 8.8284)
  line L1541 (30.8284, 11) -> (32, 12.1716)
  line L1542 (32, -1.1716) -> (30.8284, 0)
  line L1543 (30.8284, -39) -> (32, -37.8284)
  line L1544 (29.1716, -45) -> (28, -46.1716)
  line L1545 (32, -22.8284) -> (32, -21.1716)
  line L1546 (28, -26.1716) -> (28, -27.8284)
  line L1547 (28, -16.1716) -> (28, -17.8284)
  line L1548 (30.8284, -54) -> (32, -52.8284)
  line L1549 (32, -16.1716) -> (30.8284, -15)
  line L1550 (28, -11.1716) -> (28, -12.8284)
  line L1551 (29.1716, -40) -> (28, -41.1716)
  line L1552 (28, -2.8284) -> (29.1716, -4)
  line L1553 (28, -12.8284) -> (29.1716, -14)
  line L1554 (28, 3.8284) -> (28, 2.1716)
  line L1555 (32, -37.8284) -> (32, -36.1716)
  line L1556 (32, -52.8284) -> (32, -51.1716)
  line L1557 (32, -42.8284) -> (32, -41.1716)
  line L1558 (32, 3.8284) -> (30.8284, 5)
  line L1559 (30.8284, -5) -> (29.1716, -5)
  line L1560 (32, -51.1716) -> (30.8284, -50)
  line L1561 (29.1716, -30) -> (28, -31.1716)
  line L1562 (29.1716, -4) -> (30.8284, -4)
  line L1563 (32, 7.1716) -> (32, 8.8284)
  line L1564 (29.1716, -34) -> (30.8284, -34)
  line L1565 (30.8284, -15) -> (29.1716, -15)
  line L1566 (32, 2.1716) -> (32, 3.8284)
  line L1567 (30.8284, 20) -> (29.1716, 20)
  line L1568 (29.1716, -54) -> (30.8284, -54)
  line L1569 (28, 12.1716) -> (29.1716, 11)
  line L1570 (28, -36.1716) -> (28, -37.8284)
  line L1571 (32, -41.1716) -> (30.8284, -40)
  line L1572 (32, 13.8284) -> (30.8284, 15)
  line L1573 (32, 18.8284) -> (30.8284, 20)
  line L1574 (32, -7.8284) -> (32, -6.1716)
  line L1575 (30.8284, -29) -> (32, -27.8284)
  point P0 (-29, -52)
  point P1 (-29, -47)
  point P2 (-29, -42)
  point P3 (-29, -37)
  point P4 (-29, -32)
  point P5 (-29, -27)
  point P6 (-29, -22)
  point P7 (-29, -17)
  point P8 (-29, -12)
  point P9 (-29, -7)
  point P10 (-29, -2)
  point P11 (-29, 3)
  point P12 (-29, 8)
  point P13 (-29, 13)
  point P14 (-29, 18)
  point P15 (-24.0833, -27)
  point P16 (-24.0833, 18)
  point P17 (-24.0833, -32)
  point P18 (-24.0833, 13)
  point P19 (-24.0833, -52)
  point P20 (-24.0833, -17)
  point P21 (-24.0833, 3)
  point P22 (-24.0833, 8)
  point P23 (-24.0833, -7)
  point P24 (-24.0833, -22)
  point P25 (-24.0833, -12)
  point P26 (-24.0833, -42)
  point P27 (-24.0833, -2)
  point P28 (-15.2513, -43.905)
  point P29 (-24.0833, -47)
  point P30 (-24.0833, -37)
  point P31 (-19.1667, -27)
  point P32 (-19.1667, 18)
  point P33 (-19.1667, -32)
  point P34 (-19.1667, 13)
  point P35 (-19.1667, -52)
  point P36 (-19.1667, -17)
  point P37 (-19.1667, 3)
  point P38 (-19.1667, 8)
  point P39 (-19.1667, -7)
  point P40 (-19.1667, -22)
  point P41 (-19.1667, -12)
  point P42 (-19.1667, -42)
  point P43 (-19.1667, -2)
  point P44 (-10.3346, -43.905)
  point P45 (-19.1667, -47)
  point P46 (-19.1667, -37)
  point P47 (-14.25, -27)
  point P48 (-14.25, 18)
  point P49 (-14.25, -32)
  point P50 (-14.25, 13)
  point P51 (-14.25, -52)
  point P52 (-14.25, -17)
  point P53 (-14.25, 3)
  point P54 (-14.25, 8)
  point P55 (-14.25, -7)
  point P56 (-14.25, -22)
  point P57 (-14.25, -12)
  point P58 (-14.25, -42)
  point P59 (-14.25, -2)
  point P60 (-5.4179, -43.905)
  point P61 (-14.25, -47)
  point P62 (-14.25, -37)
  point P63 (-9.3333, -27)
  point P64 (-9.3333, 18)
  point P65 (-9.3333, -32)
  point P66 (-9.3333, 13)
  point P67 (-9.3333, -52)
  point P68 (-9.3333, -17)
  point P69 (-9.3333, 3)
  point P70 (-9.3333, 8)
  point P71 (-9.3333, -7)
  point P72 (-9.3333, -22)
  point P73 (-9.3333, -12)
  point P74 (-9.3333, -42)
  point P75 (-9.3333, -2)
  point P76 (-0.5013, -43.905)
  point P77 (-9.3333, -47)
  point P78 (-9.3333, -37)
  point P79 (-4.4167, -27)
  point P80 (-4.4167, 18)
  point P81 (-4.4167, -32)
  point P82 (-4.4167, 13)
  point P83 (-4.4167, -52)
  point P84 (-4.4167, -17)
  point P85 (-4.4167, 3)
  point P86 (-4.4167, 8)
  point P87 (-4.4167, -7)
  point P88 (-4.4167, -22)
  point P89 (-4.4167, -12)
  point P90 (-4.4167, -42)
  point P91 (-4.4167, -2)
  point P92 (4.4154, -43.905)
  point P93 (-4.4167, -47)
  point P94 (-4.4167, -37)
  point P95 (0.5, -27)
  point P96 (0.5, 18)
  point P97 (0.5, -32)
  point P98 (0.5, 13)
  point P99 (0.5, -52)
  point P100 (0.5, -17)
  point P101 (0.5, 3)
  point P102 (0.5, 8)
  point P103 (0.5, -7)
  point P104 (0.5, -22)
  point P105 (0.5, -12)
  point P106 (0.5, -42)
  point P107 (0.5, -2)
  point P108 (9.3321, -43.905)
  point P109 (0.5, -47)
  point P110 (0.5, -37)
  point P111 (5.4167, -27)
  point P112 (5.4167, 18)
  point P113 (5.4167, -32)
  point P114 (5.4167, 13)
  point P115 (5.4167, -52)
  point P116 (5.4167, -17)
  point P117 (5.4167, 3)
  point P118 (5.4167, 8)
  point P119 (5.4167, -7)
  point P120 (5.4167, -22)
  point P121 (5.4167, -12)
  point P122 (5.4167, -42)
  point P123 (5.4167, -2)
  point P124 (14.2487, -43.905)
  point P125 (5.4167, -47)
  point P126 (5.4167, -37)
  point P127 (10.3333, -27)
  point P128 (10.3333, 18)
  point P129 (10.3333, -32)
  point P130 (10.3333, 13)
  point P131 (10.3333, -52)
  point P132 (10.3333, -17)
  point P133 (10.3333, 3)
  point P134 (10.3333, 8)
  point P135 (10.3333, -7)
  point P136 (10.3333, -22)
  point P137 (10.3333, -12)
  point P138 (10.3333, -42)
  point P139 (10.3333, -2)
  point P140 (19.1654, -43.905)
  point P141 (10.3333, -47)
  point P142 (10.3333, -37)
  point P143 (15.25, -27)
  point P144 (15.25, 18)
  point P145 (15.25, -32)
  point P146 (15.25, 13)
  point P147 (15.25, -52)
  point P148 (15.25, -17)
  point P149 (15.25, 3)
  point P150 (15.25, 8)
  point P151 (15.25, -7)
  point P152 (15.25, -22)
  point P153 (15.25, -12)
  point P154 (15.25, -42)
  point P155 (15.25, -2)
  point P156 (24.0821, -43.905)
  point P157 (15.25, -47)
  point P158 (15.25, -37)
  point P159 (20.1667, -27)
  point P160 (20.1667, 18)
  point P161 (20.1667, -32)
  point P162 (20.1667, 13)
  point P163 (20.1667, -52)
  point P164 (20.1667, -17)
  point P165 (20.1667, 3)
  point P166 (20.1667, 8)
  point P167 (20.1667, -7)
  point P168 (20.1667, -22)
  point P169 (20.1667, -12)
  point P170 (20.1667, -42)
  point P171 (20.1667, -2)
  point P172 (28.9987, -43.905)
  point P173 (20.1667, -47)
  point P174 (20.1667, -37)
  point P175 (25.0833, -27)
  point P176 (25.0833, 18)
  point P177 (25.0833, -32)
  point P178 (25.0833, 13)
  point P179 (25.0833, -52)
  point P180 (25.0833, -17)
  point P181 (25.0833, 3)
  point P182 (25.0833, 8)
  point P183 (25.0833, -7)
  point P184 (25.0833, -22)
  point P185 (25.0833, -12)
  point P186 (25.0833, -42)
  point P187 (25.0833, -2)
  point P188 (33.9154, -43.905)
  point P189 (25.0833, -47)
  point P190 (25.0833, -37)
  point P191 (30, -27)
  point P192 (30, 18)
  point P193 (30, -32)
  point P194 (30, 13)
  point P195 (30, -52)
  point P196 (30, -17)
  point P197 (30, 3)
  point P198 (30, 8)
  point P199 (30, -7)
  point P200 (30, -22)
  point P201 (30, -12)
  point P202 (30, -42)
  point P203 (30, -2)
  point P204 (38.8321, -43.905)
  point P205 (30, -47)
  point P206 (30, -37)
  dimension "d32" = 2
  dimension "d35" = 58
  dimension "d36" = 70
  dimension "d39" = 59
  dimension "d40" = 0
  constraint horizontal L12
  constraint vertical L13
  constraint horizontal L14
  constraint vertical L15
  constraint midpoint L10 L12.start
  constraint horizontal L17
  measures "d32" distance of P0 L23
extrude "Extrude7" add sketch "Sketch6" along normal blind 1 contours L6 L7 L8 L9 L10 L12 L13 L14 L15 L16 L22 L23 L26 L29 L31 L34 L37 L39 L42 L45 L47 L50 L53 L55 L58 L61 L63 L66 L69 L71 L74 L77 L79 L82 L85 L87 L90 L93 L95 L98 L101 L103 L106 L109 L111 L114 L117 L119 L122 L125 L127 L130 L133 L135 L256 L259 L260 L262 L263 L264 L265 L275 L279 L283 L289 L292 L296 L297 L298 L302 L309 L313 L317 L320 L322 L323 L324 L325 L326 L327 L328 L334 L335 L339 L340 L346 L347 L350 L351 L352 L353 L354 L361 L369 L370 L399 L403 L448 L519 L523 L568 L639 L643 L688 L759 L763 L808 L879 L883 L928 L999 L1003 L1048 L1119 L1123 L1168 L1217 L1218 L1221 L1226 L1228 L1229 L1231 L1233 L1234 L1236 L1238 L1239 L1240 L1241 L1243 L1244 L1245 L1246 L1247 L1248 L1250 L1251 L1253 L1254 L1255 L1260 L1261 L1264 L1265 L1266 L1267 L1268 L1270 L1271 L1274 L1276 L1279 L1281 L1288 L1289 L1291 L1292 L1293 L1296 L1297 L1298 L1301 L1302 L1303 L1305 L1309 L1315 L1317 L1318 L1319 L1322 L1323 L1324 L1325 L1326 L1327 L1331 L1332 L1333 L1334 L1335 | L7 L8 L9 L12 L257 L258 L259 L261 L262 L263 L266 L268 L269 L271 L273 L274 L275 L276 L278 L279 L280 L281 L284 L285 L286 L287 L288 L289 L290 L291 L292 L293 L294 L295 L297 L298 L300 L301 L302 L304 L305 L306 L307 L308 L309 L310 L311 L314 L316 L317 L319 L321 L322 L323 L325 L326 L327 L329 L331 L332 L333 L334 L335 L336 L337 L338 L339 L340 L341 L342 L343 L345 L349 L351 L352 L353 L355 L357 L358 L359 L361 L362 L363 L364 L365 L366 L367 L369 L371 L372 L373 L374 L375 L377 L399 L444 L448 L471 L477 L491 L497 L519 L564 L568 L591 L597 L611 L617 L639 L684 L688 L711 L717 L731 L737 L759 L804 L808 L831 L837 L851 L857 L879 L924 L928 L951 L957 L971 L977 L999 L1044 L1048 L1071 L1077 L1091 L1097 L1119 L1164 L1168 L1191 L1197 L1211 L1216 L1217 L1219 L1220 L1222 L1223 L1224 L1225 L1226 L1228 L1235 L1236 L1240 L1245 L1248 L1249 L1252 L1256 L1257 L1258 L1260 L1262 L1265 L1266 L1267 L1268 L1269 L1270 L1273 L1274 L1276 L1277 L1280 L1282 L1283 L1284 L1285 L1286 L1287 L1288 L1289 L1292 L1293 L1294 L1295 L1296 L1297 L1299 L1300 L1306 L1307 L1310 L1311 L1312 L1313 L1314 L1319 L1321 L1322 L1324 L1325 L1327 L1329 L1330 | L8 L9 L328
